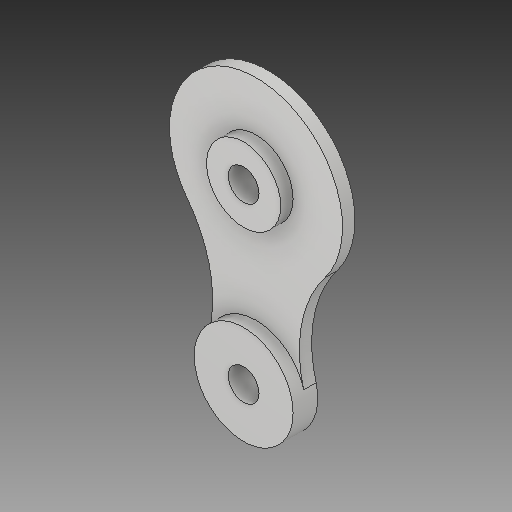
# Autodesk Inventor part: 脚揺動節抑え1
Saved by Autodesk Inventor 2020 (Build 240168000, 168)
## iProperties
Created: 2018-07-15
Part Number: 脚揺動節抑え1
Material: アルミニウム 2014-T4
Document SubType Name: Modeling
Designer: 雪村
Density: 2.8 g/cm^3
Appearance: サテン
Mass: 0.82463 g
Surface Area: 5.9116 cm^2
Volume: 0.294511 cm^3
Description: アルミ2000 2t
Author: 雪村
Autodesk Inventor part; units mm, degrees
ref_plane "YZ Plane" through (0, 0, 0) normal (1, 0, 0) x (0, 1, 0)
ref_plane "XZ Plane" through (0, 0, 0) normal (0, 1, 0) x (-1, 0, 0)
ref_plane "XY Plane" through (0, 0, 0) normal (0, 0, 1) x (1, 0, 0)
sketch "スケッチ1" plane through (0, 0, 0) normal (0, 0, 1) x (1, 0, 0)
  circle A0 centre (0, 0) radius 7
  circle A1 centre (0, -14) radius 4
  line L0 (-6.8374, -1.5) -> (-3.9071, -14.8571)
  line L1 (6.8374, -1.5) -> (3.9071, -14.8571)
  circle A2 centre (0, 0) radius 1.25
  circle A3 centre (0, -14) radius 1.25
  dimension "d0" = 14
  dimension "d1" = 8
  dimension "d2" = 14
  dimension "d3" = 2.5
  dimension "d4" = 2.5
  constraints: 4 centre point, 4 end point, 4 point on circle, 4 tangent, 3 coincident, 1 vertical alignment
  measures "d0" diameter of A0
  measures "d1" diameter of A1
  measures "d2" distance of A1.centre point (0, 0)
  measures "d3" diameter of A2
  measures "d4" diameter of A3
extrude "押し出し1" add sketch "スケッチ1" along normal blind 1
sketch "スケッチ2" plane through (0, 0, 1) normal (0, 0, 1) x (1, 0, 0)
  circle A0 centre (0, 0) radius 3
  circle A1 centre (0, 0) radius 1.25 projected
  circle A2 centre (0, -14) radius 1.25 projected
  arc A3 (-3.9071, -14.8571) -> (3.9071, -14.8571) centre (0, -14) ccw projected
  line L0 (3.9071, -14.8571) -> (6.8374, -1.5) projected
  arc A4 (6.8374, -1.5) -> (-6.8374, -1.5) centre (0, 0) ccw projected
  line L1 (-6.8374, -1.5) -> (-3.9071, -14.8571) projected
  circle A5 centre (0, -14) radius 4
  dimension "d7" = 6
  dimension "d8" = 8
  constraints: 2 centre point, 2 coincident
  measures "d7" diameter of A0
  measures "d8" diameter of A5
extrude "押し出し2" add sketch "スケッチ2" along normal blind 1 contours A0 | A5 A3
sketch "スケッチ4" plane through (0, 0, 0) normal (0, 0, -1) x (-1, 0, 0)
  circle A0 centre (0, 0) radius 1.25 projected
  circle A1 centre (0, -14) radius 1.25 projected
  arc A2 (-6.8374, -1.5) -> (-5.5621, -4.25) centre (0, 0) ccw
  arc A3 (3.9071, -14.8571) -> (3.8595, -12.949) centre (0, -14) ccw
  arc A4 (-3.8595, -12.949) -> (-5.5621, -4.25) centre (-13.5081, -10.3214) ccw
  arc A5 (5.5621, -4.25) -> (3.8595, -12.949) centre (13.5081, -10.3214) ccw
  line L0 (-3.9071, -14.8571) -> (-6.8374, -1.5) projected
  line L1 (6.8374, -1.5) -> (3.9071, -14.8571) projected
  arc A6 (-5.5621, -4.25) -> (5.5621, -4.25) centre (0, 0) ccw construction
  arc A7 (5.5621, -4.25) -> (6.8374, -1.5) centre (0, 0) ccw
  arc A8 (3.8595, -12.949) -> (-3.8595, -12.949) centre (0, -14) ccw construction
  arc A9 (-3.8595, -12.949) -> (-3.9071, -14.8571) centre (0, -14) ccw
  dimension "d15" = 10
  dimension "d16" = 10
  constraints: 18 point on circle, 8 centre point, 4 end point, 4 tangent, 2 coincident
  measures "d15" radius of A5
  measures "d16" radius of A4
extrude "押し出し3" cut sketch "スケッチ4" against normal blind 10 contours A2 A4 A9 L0 | A3 A5 A7 L1
sketch "スケッチ6" plane through (0, -14, 2) normal (0, 0, 1) x (1, 0, 0)
  arc A0 (-5.8857, 1.6028) -> (-7.2308, 8.475) centre (-13.5081, 3.6786) ccw
  arc A1 (7.2308, 8.475) -> (-7.2308, 8.475) centre (0, 14) ccw
  arc A2 (7.2308, 8.475) -> (5.8857, 1.6028) centre (13.5081, 3.6786) ccw
  arc A3 (-5.8857, 1.6028) -> (-3.8595, 1.051) centre (-4.8726, 1.3269) ccw
  arc A4 (3.8595, 1.051) -> (5.8857, 1.6028) centre (4.8726, 1.3269) ccw
  arc A5 (3.8595, 1.051) -> (-3.8595, 1.051) centre (0, 0) ccw projected
  arc A6 (-3.8595, 1.051) -> (3.8595, 1.051) centre (0, 0) ccw projected
  arc A7 (-3.8595, 1.051) -> (-5.5621, 9.75) centre (-13.5081, 3.6786) ccw projected
  arc A8 (5.5621, 9.75) -> (-5.5621, 9.75) centre (0, 14) ccw projected
  arc A9 (5.5621, 9.75) -> (3.8595, 1.051) centre (13.5081, 3.6786) ccw projected
  circle A10 centre (0, 14) radius 1.25 projected
  circle A11 centre (0, 0) radius 1.25 projected
  circle A12 centre (0, 14) radius 3 projected
  constraints: 12 point on circle, 5 centre point, 2 tangent, 5 other
